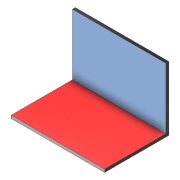
# Autodesk Inventor part: Laptop_MSI_KATANA_GF76_11UG
Saved by Autodesk Inventor 2022 (Build 260153000, 153)
## iProperties
Created: 2024-04-12
Part Number: Laptop_MSI_KATANA_GF76_11UG
Material: Generic
Document SubType Name: Modeling
Designer: LaptopJR
Density: 1 g/cm^3
Appearance: Default
Author: LaptopJR
Autodesk Inventor part; units mm, degrees
ref_plane "YZ Plane" through (0, 0, 0) normal (1, 0, 0) x (0, 1, 0)
ref_plane "XZ Plane" through (0, 0, 0) normal (0, 1, 0) x (-1, 0, 0)
ref_plane "XY Plane" through (0, 0, 0) normal (0, 0, 1) x (1, 0, 0)
sketch "Sketch2" plane through (0, 0, 0) normal (1, 0, 0) x (0, 1, 0)
  line L0 (0, 0) -> (0, -273)
  line L1 (0, -273) -> (273, -273)
  line L2 (273, -273) -> (273, -260.4)
  line L3 (273, -260.4) -> (12.6, -260.4)
  line L4 (12.6, -260.4) -> (12.6, 0)
  line L5 (12.6, 0) -> (0, 0)
  dimension "d0" = 12.6
  dimension "d1" = 12.6
  dimension "d2" = 273
  dimension "d3" = 273
  constraints: 12 end point, 4 perpendicular, 2 vertical
  measures "d0" distance of L4.end L0.start
  measures "d1" distance of L1.end L2.end
  measures "d2" distance of L0.start L0.end
  measures "d3" distance of L0.end L1.end
extrude "Extrusion1" add sketch "Sketch2" along normal blind 398
body "Solid1"
